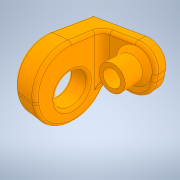
# Autodesk Inventor part: Петля ролика
Saved by Autodesk Inventor 2021.1 (Build 251245010, 245A)
## iProperties
Created: 2026-04-16
Part Number: Петля ролика
Material: Типовые
Document SubType Name: Modeling
Designer: Андрей Тарасов
Density: 1 g/cm^3
Appearance: По умолчанию
Author: Андрей Тарасов
Autodesk Inventor part; units mm, degrees
ref_plane "YZ Plane" through (0, 0, 0) normal (1, 0, 0) x (0, 1, 0)
ref_plane "XZ Plane" through (0, 0, 0) normal (0, 1, 0) x (-1, 0, 0)
ref_plane "XY Plane" through (0, 0, 0) normal (0, 0, 1) x (1, 0, 0)
sketch "Эскиз1" plane through (0, 0, 0) normal (0, 0, 1) x (1, 0, 0)
  circle A0 centre (0, 0) radius 2
  circle A1 centre (0, 0) radius 5.625 construction
  line L0 (-14, -9.625) -> (5, -9.625) construction
  line L1 (5, -9.625) -> (5, -1.625) construction
  line L2 (-14, -1.625) -> (-14, -9.625) construction
  line L3 (-14, -5.625) -> (5, -5.625) construction
  line L4 (-14, -13.625) -> (5, -13.625)
  line L5 (5, -13.625) -> (5, 5)
  line L6 (-14, 5) -> (-14, -13.625)
  circle A2 centre (0, 0) radius 6.5 construction
  line L7 (-14, 5) -> (5, 5)
  line L8 (0, -17.65) -> (0, 10.525) construction
  line L9 (-8, 5) -> (-8, -13.625) construction
  line L10 (-18.1, 0) -> (10.6, 0) construction
  line L11 (-8, -13.625) -> (-8, -6.5)
  line L12 (-8, -6.5) -> (5, -6.5)
  dimension "d0" = 4
  dimension "d1" = 11.25
  dimension "d5" = 13
  dimension "d11" = 6
  dimension "d36" = 5
  dimension "d37" = 5
  dimension "d39" = 8
  dimension "d40" = 4
  dimension "d41" = 4
  constraints: 22 end point, 4 horizontal, 4 perpendicular, 4 point on line, 3 centre point, 3 coincident, 2 collinear, 2 midpoint, 2 parallel, 2 tangent
  measures "d0" diameter of A0
  measures "d1" diameter of A1
  measures "d5" diameter of A2
  measures "d11" distance between parallel lines of L9 L6
  measures "d36" distance between parallel lines of L1 L8
  measures "d37" distance between parallel lines of L10 L7
  measures "d39" distance between parallel lines of L8 L9
  measures "d40" distance between parallel lines of L3 L0
  measures "d41" distance between parallel lines of L4 L0
extrude "Выдавливание1" add sketch "Эскиз1" along normal blind 3 contours L6 L7 L5 L12 L11 L4
sketch "Эскиз3" plane through (0, 0, 3) normal (0, 0, 1) x (1, 0, 0)
  line L0 (-14, -13.625) -> (-8, -13.625) projected
  line L1 (-14, 5) -> (-8, 5)
  line L2 (-8, 5) -> (-8, -13.625)
  line L3 (-8, -13.625) -> (-14, -13.625)
  line L4 (-14, -13.625) -> (-14, 5)
  point P0 (0, 0)
  point P1 (5, -13.625)
  point P2 (4, 5)
  dimension "d17" = 6
  constraints: 9 end point, 2 parallel, 1 horizontal, 1 perpendicular, 1 point on line
  measures "d17" distance of L1.start L1.end
extrude "Выдавливание3" add sketch "Эскиз3" along normal blind 17
sketch "Эскиз4" plane through (-14, -13.625, 0) normal (1, 0, 0) x (0, 0, -1)
  circle A0 centre (-11, 8) radius 4.3
  line L0 (0, 7.125) -> (0, 18.625) projected
  line L1 (0, 0) -> (-20, 0) projected
  line L2 (-20, 18.625) -> (-20, 0) projected
  line L3 (0, 18.625) -> (0, 0) projected
  line L4 (0, 7) -> (-6, 0)
  point P0 (0, 13.625)
  dimension "d20" = 8.6
  dimension "d42" = 9
  dimension "d48" = 8
  dimension "d49" = 7
  dimension "d50" = 6
  constraints: 2 end point, 2 point on line, 1 centre point
  measures "d20" diameter of A0
  measures "d42" distance from line of L2 A0.centre
  measures "d48" distance from line of A0.centre L1
  measures "d49" distance from line of L1 L4.start
  measures "d50" distance from line of L0 L4.end
extrude "Выдавливание4" cut sketch "Эскиз4" along normal up to surface (6 mm away)
sketch "Эскиз2" plane through (0, 0, 3) normal (0, 0, 1) x (1, 0, 0)
  circle A0 centre (0, 0) radius 3
  circle A1 centre (0, 0) radius 2 projected
  dimension "d14" = 6
  constraints: 1 centre point, 1 coincident
  measures "d14" diameter of A0
extrude "Выдавливание2" add sketch "Эскиз2" along normal blind 6
fillet "Сопряжение1" radius 9 3 edges at (-11, 5, 20) (-11, -13.625, 20) (-11, -13.625, 6)
fillet "Сопряжение1" radius 5 2 edges at (5, 5, 1.5) (5, -6.5, 1.5)
fillet "Сопряжение1" radius 2 2 edges at (-8, -6.5, 1.5) (-8, -0.75, 3)
chamfer "Фаска1" distance 1.2 angle 45 1 edges at (-3, 0, 3)
fillet "Сопряжение2" radius 0.8 9 edges at (-8, -5.625, 15.3) (-14, -5.625, 15.3) (-14, -13.625, 10.5697) (-14, 2.364, 17.364) (-8, 5, 8) (-8, -13.625, 10.5697) (-8, 2.364, 17.364) (-8, -9.4911, 2.4566) (-14, -8.5536, 1.6531)
chamfer "Фаска2" distance 0.8 angle 45 1 edges at (-2, 0, 0)
